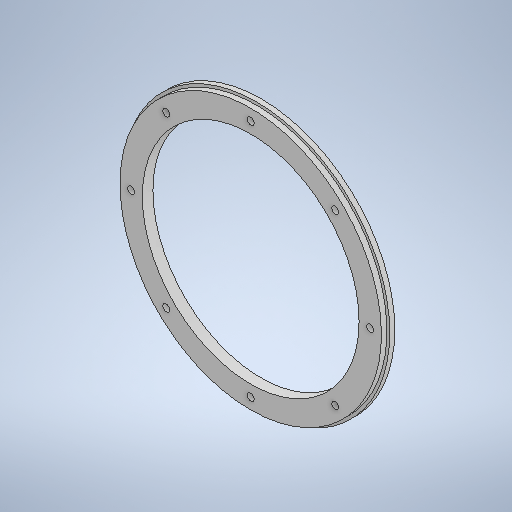
# Autodesk Inventor part: ДМФ 01 32.2 Барабан Опорное кольцо КОРМА
Saved by Autodesk Inventor 2025 (Build 290162010, 162A)
## iProperties
Created: 2024-04-28
Part Number: ДМФ 01 32.2 Барабан Опорное кольцо КОРМА
Material: Generic
Document SubType Name: Sheet Metal
Designer: admin
Density: 1 g/cm^3
Appearance: Default
Stock Number: Опорное_Кольцо_Корма
Sheet Metal Rule: Default
Flat Pattern Width: 47.9 cm
Flat Pattern Length: 47.9 cm
Flat Pattern Area: 2294.41 cm^2
Sheet Metal Width: 479,000 mm
Sheet Metal Length: 479,000 mm
Sheet Metal Area: 229441,000 mm^2
Author: pokla
Autodesk Inventor part; units mm, degrees
ref_plane "YZ Plane" through (0, 0, 0) normal (1, 0, 0) x (0, 1, 0)
ref_plane "XZ Plane" through (0, 0, 0) normal (0, 1, 0) x (-1, 0, 0)
ref_plane "XY Plane" through (0, 0, 0) normal (0, 0, 1) x (1, 0, 0)
sketch "Sketch1" plane through (0, 0, 0) normal (0, 0, 1) x (1, 0, 0)
  circle A0 centre (0, 0) radius 194.5
  circle A1 centre (0, 0) radius 234.5
  dimension "d0" = 40
  dimension "d1" = 389
  constraints: 2 centre point, 1 coincident
  measures "d0" radial gap between concentric circles of A0 A1
  measures "d1" diameter of A0
extrude "Extrusion1" add sketch "Sketch1" along normal blind 38
sketch "Sketch2" plane through (0, 0, 38) normal (0, 0, 1) x (1, 0, 0)
  circle A0 centre (0, 0) radius 234.5 construction
  circle A1 centre (0, 0) radius 194.5 construction
  line L0 (0, 234.5) -> (0, 194.5) construction
  circle A2 centre (0, 214.5) radius 6.25
  dimension "d4" = 12.5
  constraints: 3 vertical alignment, 2 end point, 1 centre point, 1 coincident, 1 midpoint, 1 vertical, 2 other
  measures "d4" diameter of A2
extrude "Extrusion2" cut sketch "Sketch2" against normal through all
sketch "Sketch3" plane through (0, 0, 38) normal (0, 0, 1) x (1, 0, 0)
  circle A0 centre (0, 214.5) radius 6.25 projected
  circle A1 centre (0, 214.5) radius 13.75
  point P0 (0, 0)
  dimension "d10" = 27.5
  constraints: 1 centre point
  measures "d10" diameter of A1
extrude "Extrusion3" cut sketch "Sketch3" against normal blind 11
pattern_circular "Circular Pattern1" count 8 over 360 about axis through (0, 0, 0) along (0, 0, 1) of "Extrusion2", "Extrusion3"
sketch "Sketch4" plane through (0, 0, 0) normal (0, 0, -1) x (-1, 0, 0)
  circle A0 centre (0, 0) radius 234.5 projected
  circle A1 centre (0, 0) radius 239.5
  dimension "d13" = 5
  constraints: 1 centre point
  measures "d13" radial gap between concentric circles of A0 A1
extrude "Extrusion4" add sketch "Sketch4" against normal blind 9
sketch "Sketch5" plane through (0, 0, 0) normal (1, 0, 0) x (0, 1, 0)
  line L0 (234.5, 9) -> (234.5, 38) projected
  line L1 (239.5, 9) -> (-239.5, 9) projected
  line L2 (239.5, 0) -> (239.5, 9) projected
  line L3 (-239.5, 0) -> (239.5, 0) projected
  line L4 (-234.5, 9) -> (-234.5, 38) projected
  line L5 (-239.5, 0) -> (-239.5, 9) projected
  line L6 (-234.5, 19) -> (234.5, 19)
  line L7 (234.5, 38) -> (-234.5, 38) projected
  line L8 (234.5, 38) -> (-234.5, 38)
  point P0 (0, 0)
  dimension "d16" = 38
  dimension "d17" = 19
  constraints: 4 end point, 2 point on line, 1 collinear, 1 perpendicular
  measures "d16" distance from line of L3 L0.end
  measures "d17" distance from line of L6 L0.end
extrude "Extrusion5" cut sketch "Sketch5" along normal through all both and the other way through all contours L6 L4 L7 L0
equation "\"d1\" = Вал_ось_диаметр_КОРМА"
equation "\"BendRadius\" = Thickness"
equation "\"BendReliefWidth\" = Thickness"
equation "\"BendReliefDepth\" = 0.5 * Thickness"
equation "\"CornerReliefSize\" = 4 * Thickness"
equation "\"MinimumRemnant\" = 2 * Thickness"
equation "\"TransitionRadius\" = BendRadius"
equation "\"JacobiRadiusSize\" = BendRadius"
equation "\"GapSize\" = Thickness"
equation "\"Вал_ось_диаметр_КОРМА\" = 389"
equation "\"Thickness\" = 19"
body "Solid1"
